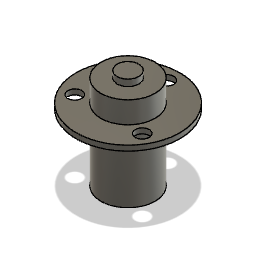
anneau coulissant rotatif v2 (Autodesk Fusion 360 design; units mm, degrees)
Autodesk Fusion 360 part; units mm, degrees
note: some values were not read from the file. Set by a fixed rule: which sketch regions a step uses.
sketch "Esquisse1" plane through (0, 0, 0) normal (0, 1, 0) x (1, 0, 0)
  circle A0 centre (0, 0) radius 12
  line L0 (0, 0) -> (0, 12)
  circle A1 centre (0, 0) radius 9
  circle A2 centre (0, 9) radius 1.6
  circle A3 centre (-7.7942, -4.5) radius 1.6
  circle A4 centre (7.7942, -4.5) radius 1.6
  dimension "d1" = 24
  dimension "d2" = 18
  dimension "d3" = 3.2
  dimension "d5" = 360
  constraint coincident A0.centre L0.start
  constraint coincident A0 L0.end
  constraint vertical L0
  constraint coincident A1 A2.centre
  constraint coincident L0 A2.centre
  measures "d1" diameter of A0
  measures "d2" diameter of A1
  measures "d3" diameter of A2
extrude "Extrusion1" add sketch "Esquisse1" along normal blind 1.2 contours A0 | A1 A2 A3 A4 makes body 1
sketch "Esquisse2" plane through (0, 1.2, 0) normal (0, 1, 0) x (-1, 0, 0)
  circle A0 centre (-7.7942, 4.5) radius 1.6
  circle A1 centre (0, -9) radius 1.6
  circle A2 centre (7.7942, 4.5) radius 1.6
  circle A3 centre (0, 0) radius 12
  circle A4 centre (0, 0) radius 6.25
  dimension "d8" = 12.5
  constraint concentric A3 A4
  measures "d8" diameter of A4
extrude "Extrusion2" add sketch "Esquisse2" along normal blind 5 contours A4 bodies 1
sketch "Esquisse3" plane through (0, 0, 0) normal (0, -1, 0) x (1, 0, 0)
  circle A0 centre (7.7942, 4.5) radius 1.6
  circle A1 centre (0, -9) radius 1.6
  circle A2 centre (-7.7942, 4.5) radius 1.6
  circle A3 centre (0, 0) radius 12
  circle A4 centre (0, 0) radius 6.25
  dimension "d11" = 12.5
  constraint concentric A3 A4
  measures "d11" diameter of A4
extrude "Extrusion3" add sketch "Esquisse3" along normal blind 15.4 contours A4 bodies 1
sketch "Esquisse4" plane through (0, 6.2, 0) normal (0, 1, 0) x (-1, 0, 0)
  circle A0 centre (0, 0) radius 6.25
  circle A1 centre (0, 0) radius 2.5
  dimension "d14" = 5
  constraint coincident A0.centre A1.centre
  measures "d14" diameter of A1
extrude "Extrusion4" add sketch "Esquisse4" along normal blind 1.5 contours A1 bodies 1
copy_body "Corps->Comp1" bodies 1 removing the originals makes body 2 in component "anneau coulissant rotatif"
component "anneau coulissant rotatif" placed x (1, 0, 0) y (0, 1, 0) z (0, 0, 1) at (0, 0, 0)
equation "d12 = 21.6 mm - 5 mm - 1.2 mm"
